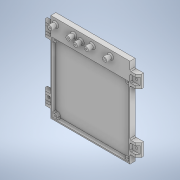
# Autodesk Inventor part: Mainboard Holder
Saved by Autodesk Inventor 2022 (Build 260153000, 153)
## iProperties
Created: 2022-04-03
Part Number: Mainboard Holder
Material: Generic
Document SubType Name: Modeling
Designer: torba
Density: 1 g/cm^3
Appearance: Default
Autodesk Inventor part; units mm, degrees
ref_plane "YZ Plane" through (0, 0, 0) normal (1, 0, 0) x (0, 1, 0)
ref_plane "XZ Plane" through (0, 0, 0) normal (0, 1, 0) x (-1, 0, 0)
ref_plane "XY Plane" through (0, 0, 0) normal (0, 0, 1) x (1, 0, 0)
sketch "0" plane through (0, 0, 0) normal (0, 0, 1) x (1, 0, 0)
  circle A0 centre (36.0915, 143.2669) radius 4
  circle A1 centre (173.2215, 143.2669) radius 4
  circle A2 centre (173.2215, 19.2669) radius 4
  circle A3 centre (36.0915, 19.2669) radius 4
  line L0 (30.0915, 13.2669) -> (179.2215, 13.2669)
  line L1 (179.2215, 13.2669) -> (179.2215, 149.2669)
  line L2 (179.2215, 149.2669) -> (30.0915, 149.2669)
  line L3 (30.0915, 149.2669) -> (30.0915, 13.2669)
  line L4 (30.0915, 149.2669) -> (179.2215, 149.2669)
  line L5 (179.2215, 149.2669) -> (179.2215, 181.2669)
  line L6 (179.2215, 181.2669) -> (30.0915, 181.2669)
  line L7 (30.0915, 181.2669) -> (30.0915, 149.2669)
  circle A4 centre (142.4715, 170.9169) radius 4
  circle A5 centre (107.9715, 170.9169) radius 4
  circle A6 centre (73.4715, 170.9169) radius 4
  circle A7 centre (38.9715, 170.9169) radius 4
  circle A8 centre (87.0915, 167.2669) radius 4
  line L8 (195.2215, 29.2669) -> (179.2215, 29.2669)
  line L9 (179.2215, 29.2669) -> (179.2215, 53.2669)
  line L10 (179.2215, 53.2669) -> (195.2215, 53.2669)
  line L11 (195.2215, 53.2669) -> (195.2215, 29.2669)
  circle A9 centre (187.2215, 41.2669) radius 2.125
  line L12 (179.2215, 34.2669) -> (195.2215, 34.2669)
  line L13 (179.2215, 48.2669) -> (195.2215, 48.2669)
  line L14 (14.0915, 53.2669) -> (30.0915, 53.2669)
  line L15 (30.0915, 48.2669) -> (14.0915, 48.2669)
  circle A10 centre (22.0915, 41.2669) radius 2.125
  line L16 (30.0915, 34.2669) -> (14.0915, 34.2669)
  line L17 (30.0915, 29.2669) -> (14.0915, 29.2669)
  line L18 (14.0915, 29.2669) -> (14.0915, 53.2669)
  line L19 (195.2215, 165.2669) -> (195.2215, 141.2669)
  line L20 (195.2215, 141.2669) -> (179.2215, 141.2669)
  line L21 (179.2215, 146.2669) -> (195.2215, 146.2669)
  circle A11 centre (187.2215, 153.2669) radius 2.125
  line L22 (179.2215, 160.2669) -> (195.2215, 160.2669)
  line L23 (179.2215, 165.2669) -> (195.2215, 165.2669)
  line L24 (14.0915, 141.2669) -> (30.0915, 141.2669)
  line L25 (30.0915, 146.2669) -> (14.0915, 146.2669)
  circle A12 centre (22.0915, 153.2669) radius 2.125
  line L26 (30.0915, 160.2669) -> (14.0915, 160.2669)
  line L27 (30.0915, 165.2669) -> (14.0915, 165.2669)
  line L28 (14.0915, 165.2669) -> (14.0915, 141.2669)
  point P0 (30.0915, 13.2669)
  point P1 (30.0915, 149.2669)
  dimension "d4" = 6
  dimension "d5" = 6
  dimension "d6" = 6
  dimension "d7" = 6
  dimension "d8" = 6
  dimension "d9" = 6
  dimension "d10" = 6
  dimension "d11" = 6
  dimension "d12" = 8.88
  dimension "d13" = 43.38
  dimension "d14" = 57
  dimension "d15" = 77.88
  dimension "d16" = 112.38
  dimension "d52" = 4.25
  dimension "d53" = 8
  dimension "d54" = 90
  dimension "d55" = 90
  dimension "d56" = 90
  dimension "d57" = 90
  dimension "d58" = 90
  dimension "d59" = 90
  dimension "d60" = 90
  dimension "d61" = 90
  dimension "d62" = 90
  dimension "d63" = 90
  dimension "d64" = 90
  dimension "d65" = 90
  dimension "d66" = 90
  dimension "d67" = 90
  dimension "d68" = 16
  dimension "d69" = 165.13
  dimension "d70" = 181.13
  dimension "d71" = 32
  dimension "d72" = 168
  dimension "d73" = 16
  dimension "d74" = 21
  dimension "d75" = 35
  dimension "d76" = 40
  dimension "d77" = 128
  dimension "d78" = 133
  dimension "d79" = 147
  dimension "d80" = 152
  dimension "d81" = 0
  dimension "d82" = 0
  dimension "d83" = 5
  dimension "d84" = 19
  dimension "d85" = 24
  dimension "d86" = 112
  dimension "d87" = 117
  dimension "d88" = 131
  dimension "d89" = 136
  dimension "d90" = 16
  dimension "d91" = 16
  dimension "d92" = 16
  dimension "d93" = 16
  dimension "d94" = 165.13
  dimension "d95" = 181.13
  dimension "d96" = 0
  dimension "d97" = 0
  dimension "d98" = 0
  dimension "d99" = 0
  dimension "d100" = 0
  dimension "d101" = 5
  dimension "d102" = 0
  constraints: 58 end point, 13 centre point, 13 parallel, 11 equal radius, 1 horizontal, 1 vertical
  measures "d4" distance from line of L0 A3.centre
  measures "d5" distance from line of L3 A3.centre
  measures "d6" distance from line of L0 A2.centre
  measures "d7" distance from line of L1 A2.centre
  measures "d8" distance from line of L2 A1.centre
  measures "d9" distance from line of L2 A0.centre
  measures "d10" distance from line of L3 A0.centre
  measures "d11" distance from line of L1 A1.centre
  measures "d12" distance from line of L7 A7.centre
  measures "d13" distance from line of L7 A6.centre
  measures "d14" distance from line of L7 A8.centre
  measures "d15" distance from line of L7 A5.centre
  measures "d16" distance from line of L7 A4.centre
  measures "d52" diameter of A11
  measures "d53" diameter of A1
  measures "d54" angle of L19 L23
  measures "d55" angle of L19 L22
  measures "d56" angle of L19 L21
  measures "d57" angle of L19 L20
  measures "d58" angle of L19 L10
  measures "d59" angle of L19 L13
  measures "d60" angle of L19 L12
  measures "d61" angle of L19 L8
  measures "d62" angle of L19 L2
  measures "d63" angle of L11 L23
  measures "d64" angle of L23 L5
  measures "d65" angle of L23 L1
  measures "d66" angle of L23 L3
  measures "d67" angle of L23 L18
  measures "d68" distance between parallel lines of L19 L9
  measures "d69" distance between parallel lines of L19 L7
  measures "d70" distance between parallel lines of L19 L28
  measures "d71" distance between parallel lines of L6 L4
  measures "d72" distance between parallel lines of L6 L0
  measures "d73" distance between parallel lines of L6 L27
  measures "d74" distance between parallel lines of L6 L26
  measures "d75" distance between parallel lines of L6 L25
  measures "d76" distance between parallel lines of L6 L24
  measures "d77" distance between parallel lines of L6 L14
  measures "d78" distance between parallel lines of L6 L15
  measures "d79" distance between parallel lines of L6 L16
  measures "d80" distance between parallel lines of L6 L17
  measures "d81" distance from line of L19.start L11
  measures "d82" distance from line of L19.start L23
  measures "d83" distance from line of L19.start L22
  measures "d84" distance from line of L19.start L21
  measures "d85" distance from line of L19.start L20
  measures "d86" distance from line of L19.start L10
  measures "d87" distance from line of L19.start L13
  measures "d88" distance from line of L19.start L12
  measures "d89" distance from line of L19.start L8
  measures "d90" distance from line of L19.start L5
  measures "d91" distance from line of L19.start L1
  measures "d92" distance from line of L19.start L6
  measures "d93" distance from line of L19.start L2
  measures "d94" distance from line of L19.start L3
  measures "d95" distance from line of L19.start L18
  measures "d96" distance from line of L23.end L19
  measures "d97" distance from line of point (195.221, 165.267) L19
  measures "d98" distance from line of point (195.221, 165.267) L23
  measures "d99" distance from line of L22.end L19
  measures "d100" distance from line of point (195.221, 160.267) L19
  measures "d101" distance from line of point (195.221, 160.267) L23
  measures "d102" distance from line of L21.end L19
extrude "Extrusion1" add sketch "0" along normal blind 2 contours L3 L2 L1 L0 | L17 L18 L16 L3 | L1 L12 L11 L8 | L15 L18 L14 L3 | L1 L10 L11 L13 | L24 L28 L25 L3 | L1 L21 L19 L20 | L7 L6 L5 L2 | L26 L28 L27 L7 | L5 L23 L19 L22
extrude "Extrusion2" add sketch "0" along normal blind 8 contours A0 | A1 | A2 | A3
extrude "Extrusion3" add sketch "0" along normal blind 20.6 contours A4 | A5 | A6 | A7 | A8
sketch "Sketch3" plane through (36.0915, 143.2669, 2) normal (0, 0, 1) x (1, 0, 0)
  circle A0 centre (0, 0) radius 4 projected
  line L0 (0, 0) -> (137.13, 0)
  line L1 (137.13, 0) -> (137.13, -124)
  line L2 (137.13, -124) -> (0, -124)
  line L3 (0, -124) -> (0, 0)
  line L4 (-3.81, 3.81) -> (140.94, 3.81)
  line L5 (140.94, 3.81) -> (140.94, -127.81)
  line L6 (140.94, -127.81) -> (-3.81, -127.81)
  line L7 (-3.81, -127.81) -> (-3.81, 3.81)
  line L8 (141.24, 4.11) -> (-4.11, 4.11)
  line L9 (-4.11, 4.11) -> (-4.11, -128.11)
  line L10 (-4.11, -128.11) -> (141.24, -128.11)
  line L11 (141.24, -128.11) -> (141.24, 4.11)
  circle A1 centre (71.88, 27.65) radius 4 projected
  circle A2 centre (106.38, 27.65) radius 4 projected
  circle A3 centre (51, 24) radius 4 projected
  circle A4 centre (2.88, 27.65) radius 4 projected
  circle A5 centre (37.38, 27.65) radius 4 projected
  circle A6 centre (0, -124) radius 4 projected
  circle A7 centre (0, 0) radius 4 projected
  circle A8 centre (137.13, -124) radius 4 projected
  circle A9 centre (137.13, 0) radius 4 projected
  line L12 (143.13, -130) -> (-6, -130) projected
  line L13 (-6, -130) -> (-6, -114) projected
  line L14 (-6, -114) -> (-22, -114) projected
  line L15 (-22, -114) -> (-22, -109) projected
  line L16 (-22, -109) -> (-6, -109) projected
  line L17 (-6, -109) -> (-6, -95) projected
  line L18 (-6, -95) -> (-22, -95) projected
  line L19 (-22, -95) -> (-22, -90) projected
  line L20 (-22, -90) -> (-6, -90) projected
  line L21 (-6, -90) -> (-6, -2) projected
  line L22 (-6, -2) -> (-22, -2) projected
  line L23 (-22, -2) -> (-22, 3) projected
  line L24 (-22, 3) -> (-6, 3) projected
  line L25 (-6, 3) -> (-6, 17) projected
  line L26 (-6, 17) -> (-22, 17) projected
  line L27 (-22, 17) -> (-22, 22) projected
  line L28 (-22, 22) -> (-6, 22) projected
  line L29 (-6, 22) -> (-6, 38) projected
  line L30 (-6, 38) -> (143.13, 38) projected
  line L31 (143.13, 38) -> (143.13, 22) projected
  line L32 (143.13, 22) -> (159.13, 22) projected
  line L33 (159.13, 22) -> (159.13, 17) projected
  line L34 (159.13, 17) -> (143.13, 17) projected
  line L35 (143.13, 17) -> (143.13, 3) projected
  line L36 (143.13, 3) -> (159.13, 3) projected
  line L37 (159.13, 3) -> (159.13, -2) projected
  line L38 (159.13, -2) -> (143.13, -2) projected
  line L39 (143.13, -2) -> (143.13, -90) projected
  line L40 (143.13, -90) -> (159.13, -90) projected
  line L41 (159.13, -90) -> (159.13, -95) projected
  line L42 (159.13, -95) -> (143.13, -95) projected
  line L43 (143.13, -95) -> (143.13, -109) projected
  line L44 (143.13, -109) -> (159.13, -109) projected
  line L45 (159.13, -109) -> (159.13, -114) projected
  line L46 (159.13, -114) -> (143.13, -114) projected
  line L47 (143.13, -114) -> (143.13, -130) projected
  point P0 (-36.0915, -143.2669)
  point P1 (1.2182, 3.81)
  point P2 (135.9118, 3.81)
  point P3 (140.94, -1.2182)
  point P4 (140.94, -122.7818)
  point P5 (135.9118, -127.81)
  point P6 (1.2182, -127.81)
  point P7 (-3.81, -122.7818)
  point P8 (-3.81, -1.2182)
  dimension "d23" = 3.81
  dimension "d24" = 124
  dimension "d25" = 137.13
  dimension "d26" = 0.3
  constraints: 24 end point, 6 parallel, 3 perpendicular, 1 horizontal, 6 other
  measures "d23" distance between parallel lines of L3 L7
  measures "d24" distance of L1.end point (137.13, 0)
  measures "d25" distance of L1.end point (0, -124)
  measures "d26" distance between parallel lines of L4 L8
extrude "Extrusion4" add sketch "Sketch3" along normal blind 7.6 contours L4 A0 | A9 L4 | A0 L7 | L7 A6 | L5 A9 | A6 L6 | A8 L5 | L6 A8 | L11 L10 L9 L8
sketch "Sketch4" plane through (0, 0, 2) normal (0, 0, 1) x (1, 0, 0)
  circle A0 centre (107.9715, 170.9169) radius 4 projected
  circle A1 centre (142.4715, 170.9169) radius 4 projected
  circle A2 centre (87.0915, 167.2669) radius 4 projected
  circle A3 centre (38.9715, 170.9169) radius 4 projected
  circle A4 centre (73.4715, 170.9169) radius 4 projected
  line L0 (179.2215, 13.2669) -> (30.0915, 13.2669) projected
  line L1 (30.0915, 13.2669) -> (30.0915, 29.2669) projected
  line L2 (30.0915, 29.2669) -> (14.0915, 29.2669) projected
  line L3 (14.0915, 29.2669) -> (14.0915, 34.2669) projected
  line L4 (14.0915, 34.2669) -> (30.0915, 34.2669) projected
  line L5 (30.0915, 34.2669) -> (30.0915, 48.2669) projected
  line L6 (30.0915, 48.2669) -> (14.0915, 48.2669) projected
  line L7 (14.0915, 48.2669) -> (14.0915, 53.2669) projected
  line L8 (14.0915, 53.2669) -> (30.0915, 53.2669) projected
  line L9 (30.0915, 53.2669) -> (30.0915, 141.2669) projected
  line L10 (30.0915, 141.2669) -> (14.0915, 141.2669) projected
  line L11 (14.0915, 141.2669) -> (14.0915, 146.2669) projected
  line L12 (14.0915, 146.2669) -> (30.0915, 146.2669) projected
  line L13 (30.0915, 146.2669) -> (30.0915, 160.2669) projected
  line L14 (30.0915, 160.2669) -> (14.0915, 160.2669) projected
  line L15 (14.0915, 160.2669) -> (14.0915, 165.2669) projected
  line L16 (14.0915, 165.2669) -> (30.0915, 165.2669) projected
  line L17 (30.0915, 165.2669) -> (30.0915, 181.2669) projected
  line L18 (30.0915, 181.2669) -> (179.2215, 181.2669) projected
  line L19 (179.2215, 181.2669) -> (179.2215, 165.2669) projected
  line L20 (179.2215, 165.2669) -> (195.2215, 165.2669) projected
  line L21 (195.2215, 165.2669) -> (195.2215, 160.2669) projected
  line L22 (195.2215, 160.2669) -> (179.2215, 160.2669) projected
  line L23 (179.2215, 160.2669) -> (179.2215, 146.2669) projected
  line L24 (179.2215, 146.2669) -> (195.2215, 146.2669) projected
  line L25 (195.2215, 146.2669) -> (195.2215, 141.2669) projected
  line L26 (195.2215, 141.2669) -> (179.2215, 141.2669) projected
  line L27 (179.2215, 141.2669) -> (179.2215, 53.2669) projected
  line L28 (179.2215, 53.2669) -> (195.2215, 53.2669) projected
  line L29 (195.2215, 53.2669) -> (195.2215, 48.2669) projected
  line L30 (195.2215, 48.2669) -> (179.2215, 48.2669) projected
  line L31 (179.2215, 48.2669) -> (179.2215, 34.2669) projected
  line L32 (179.2215, 34.2669) -> (195.2215, 34.2669) projected
  line L33 (195.2215, 34.2669) -> (195.2215, 29.2669) projected
  line L34 (195.2215, 29.2669) -> (179.2215, 29.2669) projected
  line L35 (179.2215, 29.2669) -> (179.2215, 13.2669) projected
  line L36 (31.9815, 147.3769) -> (177.3315, 147.3769) projected
  line L37 (177.3315, 147.3769) -> (177.3315, 15.1569) projected
  line L38 (177.3315, 15.1569) -> (31.9815, 15.1569) projected
  line L39 (31.9815, 15.1569) -> (31.9815, 147.3769) projected
  line L40 (172.0033, 147.0769) -> (37.3096, 147.0769) projected
  arc A5 (32.2815, 142.0487) -> (37.3096, 147.0769) centre (36.0915, 143.2669) ccw projected
  line L41 (32.2815, 142.0487) -> (32.2815, 20.485) projected
  arc A6 (37.3096, 15.4569) -> (32.2815, 20.485) centre (36.0915, 19.2669) ccw projected
  line L42 (37.3096, 15.4569) -> (172.0033, 15.4569) projected
  arc A7 (177.0315, 20.485) -> (172.0033, 15.4569) centre (173.2215, 19.2669) ccw projected
  line L43 (177.0315, 20.485) -> (177.0315, 142.0487) projected
  arc A8 (172.0033, 147.0769) -> (177.0315, 142.0487) centre (173.2215, 143.2669) ccw projected
  line L44 (32.2815, 15.4569) -> (34.8733, 15.4569) projected
  arc A9 (32.2815, 18.0487) -> (34.8733, 15.4569) centre (36.0915, 19.2669) ccw projected
  line L45 (32.2815, 18.0487) -> (32.2815, 15.4569) projected
  line L46 (174.4396, 15.4569) -> (177.0315, 15.4569) projected
  line L47 (177.0315, 15.4569) -> (177.0315, 18.0487) projected
  arc A10 (174.4396, 15.4569) -> (177.0315, 18.0487) centre (173.2215, 19.2669) ccw projected
  line L48 (32.2815, 147.0769) -> (32.2815, 144.485) projected
  arc A11 (34.8733, 147.0769) -> (32.2815, 144.485) centre (36.0915, 143.2669) ccw projected
  line L49 (34.8733, 147.0769) -> (32.2815, 147.0769) projected
  line L50 (177.0315, 147.0769) -> (174.4396, 147.0769) projected
  arc A12 (177.0315, 144.485) -> (174.4396, 147.0769) centre (173.2215, 143.2669) ccw projected
  line L51 (177.0315, 144.485) -> (177.0315, 147.0769) projected
  point P0 (0, 0)
extrude "Extrusion5" add sketch "Sketch4" along normal up to surface (7.6 mm away) contours L0 L1 L2 L3 L4 L5 L6 L7 L8 L9 L10 L11 L12 L13 L14 L15 L16 L17 L18 L19 L20 L21 L22 L23 L24 L25 L26 L27 L28 L29 L30 L31 L32 L33 L34 L35
sketch "Sketch5" plane through (0, 0, 2) normal (0, 0, 1) x (1, 0, 0)
  line L0 (32.2815, 15.4569) -> (34.8733, 15.4569) projected
  arc A0 (32.2815, 18.0487) -> (34.8733, 15.4569) centre (36.0915, 19.2669) ccw projected
  line L1 (32.2815, 18.0487) -> (32.2815, 15.4569) projected
  line L2 (174.4396, 15.4569) -> (177.0315, 15.4569) projected
  line L3 (177.0315, 15.4569) -> (177.0315, 18.0487) projected
  arc A1 (174.4396, 15.4569) -> (177.0315, 18.0487) centre (173.2215, 19.2669) ccw projected
  line L4 (32.2815, 147.0769) -> (32.2815, 144.485) projected
  arc A2 (34.8733, 147.0769) -> (32.2815, 144.485) centre (36.0915, 143.2669) ccw projected
  line L5 (34.8733, 147.0769) -> (32.2815, 147.0769) projected
  line L6 (177.0315, 147.0769) -> (174.4396, 147.0769) projected
  arc A3 (177.0315, 144.485) -> (174.4396, 147.0769) centre (173.2215, 143.2669) ccw projected
  line L7 (177.0315, 144.485) -> (177.0315, 147.0769) projected
  line L8 (177.0315, 20.485) -> (177.0315, 142.0487) projected
  arc A4 (172.0033, 147.0769) -> (177.0315, 142.0487) centre (173.2215, 143.2669) ccw projected
  line L9 (172.0033, 147.0769) -> (37.3096, 147.0769) projected
  arc A5 (32.2815, 142.0487) -> (37.3096, 147.0769) centre (36.0915, 143.2669) ccw projected
  line L10 (32.2815, 142.0487) -> (32.2815, 20.485) projected
  arc A6 (37.3096, 15.4569) -> (32.2815, 20.485) centre (36.0915, 19.2669) ccw projected
  line L11 (37.3096, 15.4569) -> (172.0033, 15.4569) projected
  arc A7 (177.0315, 20.485) -> (172.0033, 15.4569) centre (173.2215, 19.2669) ccw projected
  line L12 (179.2215, 13.2669) -> (30.0915, 13.2669) projected
  line L13 (30.0915, 13.2669) -> (30.0915, 29.2669) projected
  line L14 (30.0915, 29.2669) -> (14.0915, 29.2669) projected
  line L15 (14.0915, 29.2669) -> (14.0915, 34.2669) projected
  line L16 (14.0915, 34.2669) -> (30.0915, 34.2669) projected
  line L17 (30.0915, 34.2669) -> (30.0915, 48.2669) projected
  line L18 (30.0915, 48.2669) -> (14.0915, 48.2669) projected
  line L19 (14.0915, 48.2669) -> (14.0915, 53.2669) projected
  line L20 (14.0915, 53.2669) -> (30.0915, 53.2669) projected
  line L21 (30.0915, 53.2669) -> (30.0915, 141.2669) projected
  line L22 (30.0915, 141.2669) -> (14.0915, 141.2669) projected
  line L23 (14.0915, 141.2669) -> (14.0915, 146.2669) projected
  line L24 (14.0915, 146.2669) -> (30.0915, 146.2669) projected
  line L25 (30.0915, 146.2669) -> (30.0915, 160.2669) projected
  line L26 (30.0915, 160.2669) -> (14.0915, 160.2669) projected
  line L27 (14.0915, 160.2669) -> (14.0915, 165.2669) projected
  line L28 (14.0915, 165.2669) -> (30.0915, 165.2669) projected
  line L29 (30.0915, 165.2669) -> (30.0915, 181.2669) projected
  line L30 (30.0915, 181.2669) -> (179.2215, 181.2669) projected
  line L31 (179.2215, 181.2669) -> (179.2215, 165.2669) projected
  line L32 (179.2215, 165.2669) -> (195.2215, 165.2669) projected
  line L33 (195.2215, 165.2669) -> (195.2215, 160.2669) projected
  line L34 (195.2215, 160.2669) -> (179.2215, 160.2669) projected
  line L35 (179.2215, 160.2669) -> (179.2215, 146.2669) projected
  line L36 (179.2215, 146.2669) -> (195.2215, 146.2669) projected
  line L37 (195.2215, 146.2669) -> (195.2215, 141.2669) projected
  line L38 (195.2215, 141.2669) -> (179.2215, 141.2669) projected
  line L39 (179.2215, 141.2669) -> (179.2215, 53.2669) projected
  line L40 (179.2215, 53.2669) -> (195.2215, 53.2669) projected
  line L41 (195.2215, 53.2669) -> (195.2215, 48.2669) projected
  line L42 (195.2215, 48.2669) -> (179.2215, 48.2669) projected
  line L43 (179.2215, 48.2669) -> (179.2215, 34.2669) projected
  line L44 (179.2215, 34.2669) -> (195.2215, 34.2669) projected
  line L45 (195.2215, 34.2669) -> (195.2215, 29.2669) projected
  line L46 (195.2215, 29.2669) -> (179.2215, 29.2669) projected
  line L47 (179.2215, 29.2669) -> (179.2215, 13.2669) projected
  point P0 (0, 0)
extrude "Extrusion6" add sketch "Sketch5" along normal up to surface (6 mm away) contours L1 A0 L0 | A1 L3 L2 | L5 A2 L4 | L7 A3 L6
sketch "Sketch6" plane through (38.9715, 170.9169, 20.6) normal (0, 0, 1) x (1, 0, 0)
  circle A0 centre (69, 0) radius 4 projected
  circle A1 centre (103.5, 0) radius 4 projected
  circle A2 centre (48.12, -3.65) radius 4 projected
  circle A3 centre (0, 0) radius 4 projected
  circle A4 centre (34.5, 0) radius 4 projected
  circle A5 centre (0, 0) radius 1.25
  circle A6 centre (34.5, 0) radius 1.25
  circle A7 centre (48.12, -3.65) radius 1.25
  circle A8 centre (69, 0) radius 1.25
  circle A9 centre (103.5, 0) radius 1.25
  point P0 (-38.9715, -170.9169)
  dimension "d33" = 2.5
  dimension "d34" = 2.5
  dimension "d35" = 2.5
  dimension "d36" = 2.5
  dimension "d37" = 2.5
  constraints: 5 centre point, 5 coincident
  measures "d33" diameter of A5
  measures "d34" diameter of A6
  measures "d35" diameter of A7
  measures "d36" diameter of A8
  measures "d37" diameter of A9
extrude "Extrusion7" cut sketch "Sketch6" against normal blind 20.6 contours A5 | A6 | A7 | A8 | A9
sketch "Sketch7" plane through (0, 0, 8) normal (0, 0, 1) x (1, 0, 0)
  circle A0 centre (87.0915, 167.2669) radius 1.25 projected
  circle A1 centre (107.9715, 170.9169) radius 1.25 projected
  circle A2 centre (73.4715, 170.9169) radius 1.25 projected
  circle A3 centre (142.4715, 170.9169) radius 1.25 projected
  circle A4 centre (38.9715, 170.9169) radius 1.25 projected
  line L0 (177.0315, 147.0769) -> (172.0033, 147.0769) projected
  line L1 (172.0033, 147.0769) -> (37.3096, 147.0769) projected
  line L2 (37.3096, 147.0769) -> (32.2815, 147.0769) projected
  line L3 (32.2815, 147.0769) -> (32.2815, 142.0487) projected
  arc A5 (32.2815, 142.0487) -> (37.3096, 147.0769) centre (36.0915, 143.2669) ccw projected
  line L4 (177.0315, 142.0487) -> (177.0315, 147.0769) projected
  line L5 (177.0315, 20.485) -> (177.0315, 142.0487) projected
  line L6 (177.0315, 15.4569) -> (177.0315, 20.485) projected
  line L7 (172.0033, 15.4569) -> (177.0315, 15.4569) projected
  line L8 (37.3096, 15.4569) -> (172.0033, 15.4569) projected
  line L9 (32.2815, 15.4569) -> (37.3096, 15.4569) projected
  line L10 (32.2815, 20.485) -> (32.2815, 15.4569) projected
  arc A6 (37.3096, 15.4569) -> (32.2815, 20.485) centre (36.0915, 19.2669) ccw projected
  arc A7 (172.0033, 147.0769) -> (177.0315, 142.0487) centre (173.2215, 143.2669) ccw projected
  line L11 (32.2815, 142.0487) -> (32.2815, 20.485) projected
  arc A8 (177.0315, 20.485) -> (172.0033, 15.4569) centre (173.2215, 19.2669) ccw projected
  line L12 (179.2215, 13.2669) -> (30.0915, 13.2669) projected
  line L13 (30.0915, 13.2669) -> (30.0915, 29.2669) projected
  line L14 (30.0915, 29.2669) -> (14.0915, 29.2669) projected
  line L15 (14.0915, 29.2669) -> (14.0915, 34.2669) projected
  line L16 (14.0915, 34.2669) -> (30.0915, 34.2669) projected
  line L17 (30.0915, 34.2669) -> (30.0915, 48.2669) projected
  line L18 (30.0915, 48.2669) -> (14.0915, 48.2669) projected
  line L19 (14.0915, 48.2669) -> (14.0915, 53.2669) projected
  line L20 (14.0915, 53.2669) -> (30.0915, 53.2669) projected
  line L21 (30.0915, 53.2669) -> (30.0915, 141.2669) projected
  line L22 (30.0915, 141.2669) -> (14.0915, 141.2669) projected
  line L23 (14.0915, 141.2669) -> (14.0915, 146.2669) projected
  line L24 (14.0915, 146.2669) -> (30.0915, 146.2669) projected
  line L25 (30.0915, 146.2669) -> (30.0915, 160.2669) projected
  line L26 (30.0915, 160.2669) -> (14.0915, 160.2669) projected
  line L27 (14.0915, 160.2669) -> (14.0915, 165.2669) projected
  line L28 (14.0915, 165.2669) -> (30.0915, 165.2669) projected
  line L29 (30.0915, 165.2669) -> (30.0915, 181.2669) projected
  line L30 (30.0915, 181.2669) -> (179.2215, 181.2669) projected
  line L31 (179.2215, 181.2669) -> (179.2215, 165.2669) projected
  line L32 (179.2215, 165.2669) -> (195.2215, 165.2669) projected
  line L33 (195.2215, 165.2669) -> (195.2215, 160.2669) projected
  line L34 (195.2215, 160.2669) -> (179.2215, 160.2669) projected
  line L35 (179.2215, 160.2669) -> (179.2215, 146.2669) projected
  line L36 (179.2215, 146.2669) -> (195.2215, 146.2669) projected
  line L37 (195.2215, 146.2669) -> (195.2215, 141.2669) projected
  line L38 (195.2215, 141.2669) -> (179.2215, 141.2669) projected
  line L39 (179.2215, 141.2669) -> (179.2215, 53.2669) projected
  line L40 (179.2215, 53.2669) -> (195.2215, 53.2669) projected
  line L41 (195.2215, 53.2669) -> (195.2215, 48.2669) projected
  line L42 (195.2215, 48.2669) -> (179.2215, 48.2669) projected
  line L43 (179.2215, 48.2669) -> (179.2215, 34.2669) projected
  line L44 (179.2215, 34.2669) -> (195.2215, 34.2669) projected
  line L45 (195.2215, 34.2669) -> (195.2215, 29.2669) projected
  line L46 (195.2215, 29.2669) -> (179.2215, 29.2669) projected
  line L47 (179.2215, 29.2669) -> (179.2215, 13.2669) projected
  circle A9 centre (173.2215, 143.2669) radius 1.25
  arc A10 (177.0315, 20.485) -> (172.0033, 15.4569) centre (173.2215, 19.2669) ccw projected
  circle A11 centre (173.2215, 19.2669) radius 1.25
  circle A12 centre (36.0915, 143.2669) radius 1.25
  circle A13 centre (36.0915, 19.2669) radius 1.25
  point P0 (0, 0)
  dimension "d40" = 2.5
  dimension "d41" = 2.5
  dimension "d42" = 2.5
  dimension "d43" = 2.5
  constraints: 4 centre point, 4 coincident
  measures "d40" diameter of A9
  measures "d41" diameter of A11
  measures "d42" diameter of A12
  measures "d43" diameter of A13
extrude "Extrusion8" cut sketch "Sketch7" against normal blind 20.6 contours A9 | A11 | A12 | A13
extrude "Extrusion9" add sketch "0" along normal blind 5 contours L16 L18 L15 L3 | L1 L13 L11 L12 | L25 L28 L26 L7 L3 | L1 L5 L22 L19 L21
chamfer "Chamfer1" distance 6 angle 45 5 edges at (14.0915, 162.7669, 9.6) (14.0915, 143.7669, 9.6) (14.0915, 50.7669, 9.6) (195.2215, 31.7669, 9.6) (195.2215, 143.7669, 9.6)
fillet "Fillet1" radius 2 29 edges at (30.0915, 160.2669, 7.3) (30.0915, 146.2669, 7.3) (30.0915, 141.2669, 4.8) (30.0915, 165.2669, 4.8) (30.0915, 53.2669, 4.8) (30.0915, 34.2669, 7.3) (30.0915, 29.2669, 4.8) (30.0915, 48.2669, 7.3) (179.2215, 29.2669, 4.8) (179.2215, 53.2669, 4.8) (179.2215, 48.2669, 7.3) (179.2215, 34.2669, 7.3) (179.2215, 141.2669, 4.8) (179.2215, 146.2669, 7.3) (179.2215, 160.2669, 7.3) (179.2215, 165.2669, 4.8) (177.0315, 142.0487, 5) (172.0033, 147.0769, 5) (172.0033, 15.4569, 5) (177.0315, 20.485, 5) (37.3096, 15.4569, 5) (32.2815, 20.485, 5) (37.3096, 147.0769, 5) (32.2815, 142.0487, 5) (34.9715, 170.9169, 9.6) (69.4715, 170.9169, 9.6) (83.0915, 167.2669, 9.6) (103.9715, 170.9169, 9.6) (138.4715, 170.9169, 9.6)
sketch "Sketch8" plane through (0, 0, 0) normal (0, 0, -1) x (-1, 0, 0)
  arc A0 (-28.0915, 141.2669) -> (-30.0915, 139.2669) centre (-28.0915, 139.2669) ccw projected
  line L0 (-30.0915, 139.2669) -> (-30.0915, 55.2669) projected
  arc A1 (-30.0915, 55.2669) -> (-28.0915, 53.2669) centre (-28.0915, 55.2669) ccw projected
  line L1 (-28.0915, 53.2669) -> (-14.0915, 53.2669) projected
  line L2 (-14.0915, 53.2669) -> (-14.0915, 29.2669) projected
  line L3 (-14.0915, 29.2669) -> (-28.0915, 29.2669) projected
  arc A2 (-28.0915, 29.2669) -> (-30.0915, 27.2669) centre (-28.0915, 27.2669) ccw projected
  line L4 (-30.0915, 27.2669) -> (-30.0915, 13.2669) projected
  line L5 (-30.0915, 13.2669) -> (-179.2215, 13.2669) projected
  line L6 (-179.2215, 13.2669) -> (-179.2215, 27.2669) projected
  arc A3 (-179.2215, 27.2669) -> (-181.2215, 29.2669) centre (-181.2215, 27.2669) ccw projected
  line L7 (-181.2215, 29.2669) -> (-195.2215, 29.2669) projected
  line L8 (-195.2215, 29.2669) -> (-195.2215, 53.2669) projected
  line L9 (-195.2215, 53.2669) -> (-181.2215, 53.2669) projected
  arc A4 (-181.2215, 53.2669) -> (-179.2215, 55.2669) centre (-181.2215, 55.2669) ccw projected
  line L10 (-179.2215, 55.2669) -> (-179.2215, 139.2669) projected
  arc A5 (-179.2215, 139.2669) -> (-181.2215, 141.2669) centre (-181.2215, 139.2669) ccw projected
  line L11 (-181.2215, 141.2669) -> (-195.2215, 141.2669) projected
  line L12 (-195.2215, 141.2669) -> (-195.2215, 165.2669) projected
  line L13 (-195.2215, 165.2669) -> (-181.2215, 165.2669) projected
  arc A6 (-181.2215, 165.2669) -> (-179.2215, 167.2669) centre (-181.2215, 167.2669) ccw projected
  line L14 (-179.2215, 167.2669) -> (-179.2215, 181.2669) projected
  line L15 (-179.2215, 181.2669) -> (-30.0915, 181.2669) projected
  line L16 (-30.0915, 181.2669) -> (-30.0915, 167.2669) projected
  arc A7 (-30.0915, 167.2669) -> (-28.0915, 165.2669) centre (-28.0915, 167.2669) ccw projected
  line L17 (-28.0915, 165.2669) -> (-14.0915, 165.2669) projected
  line L18 (-14.0915, 165.2669) -> (-14.0915, 141.2669) projected
  line L19 (-14.0915, 141.2669) -> (-28.0915, 141.2669) projected
  circle A8 centre (-187.2215, 153.2669) radius 2.125 projected
  circle A9 centre (-22.0915, 41.2669) radius 2.125 projected
  circle A10 centre (-187.2215, 41.2669) radius 2.125 projected
  circle A11 centre (-22.0915, 153.2669) radius 2.125 projected
  circle A12 centre (-173.2215, 19.2669) radius 1.25 projected
  circle A13 centre (-173.2215, 143.2669) radius 1.25 projected
  circle A14 centre (-36.0915, 19.2669) radius 1.25 projected
  circle A15 centre (-36.0915, 143.2669) radius 1.25 projected
  circle A16 centre (-87.0915, 167.2669) radius 1.25 projected
  circle A17 centre (-107.9715, 170.9169) radius 1.25 projected
  circle A18 centre (-73.4715, 170.9169) radius 1.25 projected
  circle A19 centre (-142.4715, 170.9169) radius 1.25 projected
  circle A20 centre (-38.9715, 170.9169) radius 1.25 projected
  point P0 (0, 0)
  dimension "d244" = 0
extrude "Extrusion10" add sketch "Sketch8" against normal blind 0.5 contours A0 L0 A1 L1 L2 L3 A2 L4 L5 L6 A3 L7 L8 L9 A4 L10 A5 L11 L12 L13 A6 L14 L15 L16 A7 L17 L18 L19 | A12 | A13 | A14 | A15 | A16 | A17 | A18 | A19 | A20
equation "\"d34\" = d33"
equation "\"d35\" = d33"
equation "\"d36\" = d33"
equation "\"d37\" = d33"
equation "\"d41\" = d40"
equation "\"d42\" = d40"
equation "\"d43\" = d40"
body "Solid1"
